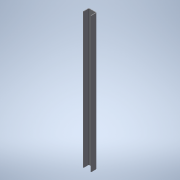
# Autodesk Inventor part: SP32V1 Refuerzo
Saved by Autodesk Inventor 2021.2 (Build 252289000, 289)
## iProperties
Created: 2026-08-14
Part Number: SP32V1 Refuerzo
Material: Generic
Document SubType Name: Sheet Metal
Designer: nelso
Density: 1 g/cm^3
Sheet Metal Rule: Default_mm
Appearance: Default
Author: nelso
Autodesk Inventor part; units mm, degrees
ref_plane "YZ Plane" through (0, 0, 0) normal (1, 0, 0) x (0, 1, 0)
ref_plane "XZ Plane" through (0, 0, 0) normal (0, 1, 0) x (-1, 0, 0)
ref_plane "XY Plane" through (0, 0, 0) normal (0, 0, 1) x (1, 0, 0)
sketch "Sketch1" plane through (0, 0, 0) normal (0, 1, 0) x (-1, 0, 0)
  line L0 (-16, 375) -> (16, 375)
  line L1 (16, 375) -> (16, -375)
  line L2 (16, -375) -> (-16, -375)
  line L3 (-16, -375) -> (-16, 375)
  line L4 (-16, 375) -> (16, -375) construction
  line L5 (16, 375) -> (-16, -375) construction
  point P0 (0, 0)
  dimension "d0" = 32
  dimension "d1" = 750
  measures "d0" distance of L1.end L2.end
  measures "d1" distance of L0.end L1.end
extrude "Plate1" add sketch "Sketch1" along normal blind 3.2
sketch "Sketch2" plane through (19.2, -3.2, 375) normal (1, 0, 0) x (0, 1, 0)
  line L0 (0, -750) -> (0, 0)
  line L1 (0, 0) -> (-25.6, 0)
  line L2 (-25.6, 0) -> (-25.6, -750)
  line L3 (-25.6, -750) -> (0, -750)
  constraints: 6 end point, 1 horizontal, 1 perpendicular, 1 vertical
edge flange "Flange1" height 32 angle 90 thickness 3.2 bend radius 3.2 thickness toward (1, 0, 0) relief straight relief width 3.2 relief depth 1.6 corner gap 3.2 corner form 0 edges at (16, 0, 0) (-16, 0, 0) wall of the first edge with corners at (19.2, -3.2, -375) (19.2, -3.2, 375) (19.2, -28.8, 375) (19.2, -28.8, -375)
bend "Bend1"
corner "Corner1"
sketch "Sketch3" plane through (0, 0, 0) normal (0, -1, 0) x (1, 0, 0)
  circle A0 centre (7, 362.3943) radius 3.3 projected
  circle A1 centre (-7, 362.3943) radius 3.3 projected
  line L0 (14, 383.091) -> (-14, 383.091) projected
  line L1 (-14, 355.3943) -> (-14, 383.091) projected
  line L2 (-14, 355.3943) -> (14, 355.3943) projected
  line L3 (14, 383.091) -> (14, 355.3943) projected
  point P0 (0, 0)
cut "Cut1" [suppressed]
equation "\"d13\" = Thickness"
equation "\"d2\" = Thickness"
equation "\"d3\" = BendReliefWidth"
equation "\"d4\" = BendReliefDepth"
equation "\"d5\" = MinimumRemnant"
equation "\"d6\" = TransitionRadius"
equation "\"d9\" = BendRadius"
equation "\"d10\" = CornerReliefSize"
equation "\"d11\" = GapSize"
equation "\"d12\" = JacobiRadiusSize"
equation "\"BendRadius\" = Thickness"
equation "\"BendReliefWidth\" = Thickness"
equation "\"BendReliefDepth\" = 0.5 * Thickness"
equation "\"CornerReliefSize\" = 4 * Thickness"
equation "\"MinimumRemnant\" = 2 * Thickness"
equation "\"TransitionRadius\" = BendRadius"
equation "\"JacobiRadiusSize\" = BendRadius"
equation "\"GapSize\" = Thickness"
equation "\"Thickness\" = 3.2"
body "Solid1"
